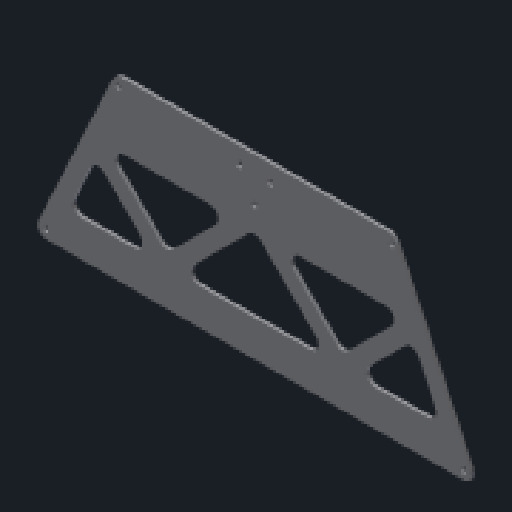
# Autodesk Inventor part: ChestFront
Saved by Autodesk Inventor 2025.2 (Build 292293000, 293)
## iProperties
Created: 2025-02-22
Part Number: ChestFront
Material: Generic
Document SubType Name: Sheet Metal
Designer: valer
Density: 1 g/cm^3
Sheet Metal Rule: Default
Appearance: Default
Author: valer
Autodesk Inventor part; units mm, degrees
ref_plane "YZ Plane" through (0, 0, 0) normal (1, 0, 0) x (0, 1, 0)
ref_plane "XZ Plane" through (0, 0, 0) normal (0, 1, 0) x (-1, 0, 0)
ref_plane "XY Plane" through (0, 0, 0) normal (0, 0, 1) x (1, 0, 0)
sketch "Sketch1" plane through (0, 0, 0) normal (0, 0, 1) x (1, 0, 0)
  line L0 (-64.749, 104.525) -> (-139.8022, 4.926) construction
  line L1 (0, 104.525) -> (-64.749, 104.525) construction
  line L2 (-139.8022, 4.926) -> (-218.9225, -165.525) construction
  line L3 (0, -219.535) -> (0, 158.535) construction
  line L4 (64.749, 104.525) -> (139.8022, 4.926) construction
  line L5 (0, 104.525) -> (64.749, 104.525) construction
  line L6 (139.8022, 4.926) -> (218.9225, -165.525) construction
  line L7 (-218.9225, -165.525) -> (0, -165.525) construction
  line L8 (218.9225, -165.525) -> (0, -165.525) construction
  line L9 (-62.7547, 100.525) -> (-136.3525, 2.8574) construction
  line L10 (-136.3525, 2.8574) -> (-212.6558, -161.525)
  line L11 (-212.6558, -161.525) -> (0, -161.525)
  line L12 (0, -161.525) -> (212.6558, -161.525)
  line L13 (212.6558, -161.525) -> (136.3525, 2.8574)
  line L14 (136.3525, 2.8574) -> (62.7547, 100.525) construction
  line L15 (62.7547, 100.525) -> (0, 100.525) construction
  line L16 (0, 100.525) -> (-62.7547, 100.525) construction
  line L17 (-136.3525, 2.8574) -> (-131.8312, 8.8574)
  line L18 (-131.8312, 8.8574) -> (0, 8.8574)
  line L19 (136.3525, 2.8574) -> (131.8312, 8.8574)
  line L20 (131.8312, 8.8574) -> (0, 8.8574)
  point P0 (0, 0)
  dimension "d0" = 4
  dimension "d34" = 6
  measures "d0" distance between parallel lines of L1 L16
  measures "d34" distance from line of L18 L9.end
extrude "Plate1" add sketch "Sketch1" along normal blind 3.048
fillet "Fillet1" radius 8 6 edges at (-212.6558, -161.525, 1.524) (212.6558, -161.525, 1.524) (-131.8312, 8.8574, 1.524) (-136.3525, 2.8574, 1.524) (131.8312, 8.8574, 1.524) (136.3525, 2.8574, 1.524)
sketch "Sketch3" plane through (0, 0, 3.048) normal (0, 0, 1) x (1, 0, 0)
  arc A0 (200.1225, -161.525) -> (207.3789, -150.1567) centre (200.1225, -153.525) ccw construction
  line L0 (136.7095, 2.0883) -> (207.3789, -150.1567) construction
  line L1 (-207.3789, -150.1567) -> (-136.7095, 2.0883) construction
  arc A1 (-207.3789, -150.1567) -> (-200.1225, -161.525) centre (-200.1225, -153.525) ccw construction
  line L2 (200.1225, -161.525) -> (-200.1225, -161.525) construction
  line L3 (-59.7632, 94.525) -> (59.7632, 94.525) construction
  line L4 (59.7632, 94.525) -> (131.178, -0.2457) construction
  line L5 (131.178, -0.2457) -> (203.2558, -155.525) construction
  line L6 (203.2558, -155.525) -> (-203.2558, -155.525) construction
  line L7 (-203.2558, -155.525) -> (-131.178, -0.2457) construction
  line L8 (-131.178, -0.2457) -> (-59.7632, 94.525) construction
  circle A2 centre (-59.7632, 94.525) radius 3
  circle A3 centre (59.7632, 94.525) radius 3
  circle A4 centre (-131.178, -0.2457) radius 3
  circle A5 centre (131.178, -0.2457) radius 3
  circle A6 centre (-200.1225, -153.525) radius 3
  line L9 (0, -215.7211) -> (0, 149.7327) construction
  circle A7 centre (200.1225, -153.525) radius 3
  arc A8 (136.7095, 2.0883) -> (135.8422, 3.5345) centre (129.4531, -1.28) ccw projected
  line L10 (134.2316, 5.6719) -> (135.8422, 3.5345) projected
  arc A9 (134.2316, 5.6719) -> (127.8425, 8.8574) centre (127.8425, 0.8574) ccw projected
  line L11 (-127.8425, 8.8574) -> (127.8425, 8.8574) projected
  arc A10 (-127.8425, 8.8574) -> (-134.2316, 5.6719) centre (-127.8425, 0.8574) ccw projected
  line L12 (-135.8422, 3.5345) -> (-134.2316, 5.6719) projected
  arc A11 (-135.8422, 3.5345) -> (-136.7095, 2.0883) centre (-129.4531, -1.28) ccw projected
  point P0 (0, 0)
  dimension "d4" = 6
  constraints: 12 end point, 6 centre point, 5 coincident, 4 equal radius, 1 symmetric about line, 3 other
  measures "d4" diameter of A2
extrude "Cut1" cut sketch "Sketch3" against normal blind 3.048
sketch "Sketch5" plane through (0, 0, 3.048) normal (0, 0, 1) x (1, 0, 0)
  circle A0 centre (-131.178, -0.2457) radius 3 construction
  circle A1 centre (131.178, -0.2457) radius 3 construction
  circle A2 centre (-200.1225, -153.525) radius 3 construction
  circle A3 centre (200.1225, -153.525) radius 3 construction
  arc A4 (136.7095, 2.0883) -> (135.8422, 3.5345) centre (129.4531, -1.28) ccw construction
  line L0 (134.2316, 5.6719) -> (135.8422, 3.5345) construction
  arc A5 (134.2316, 5.6719) -> (127.8425, 8.8574) centre (127.8425, 0.8574) ccw construction
  line L1 (-127.8425, 8.8574) -> (127.8425, 8.8574) construction
  arc A6 (-127.8425, 8.8574) -> (-134.2316, 5.6719) centre (-127.8425, 0.8574) ccw construction
  line L2 (-135.8422, 3.5345) -> (-134.2316, 5.6719) construction
  arc A7 (-135.8422, 3.5345) -> (-136.7095, 2.0883) centre (-129.4531, -1.28) ccw construction
  line L3 (-207.3789, -150.1567) -> (-136.7095, 2.0883) construction
  arc A8 (-207.3789, -150.1567) -> (-200.1225, -161.525) centre (-200.1225, -153.525) ccw construction
  line L4 (200.1225, -161.525) -> (-200.1225, -161.525) construction
  arc A9 (200.1225, -161.525) -> (207.3789, -150.1567) centre (200.1225, -153.525) ccw construction
  line L5 (136.7095, 2.0883) -> (207.3789, -150.1567) construction
  line L6 (0, -198.138) -> (0, 44.2342) construction
  line L7 (-100, 8.8574) -> (-100, -161.525) construction
  line L8 (-207.3789, -150.1567) -> (-136.7095, 2.0883) projected
  line L9 (200.1225, -161.525) -> (-200.1225, -161.525) projected
  line L10 (-15, -7.1426) -> (15, -7.1426) construction
  line L11 (15, -7.1426) -> (0, -33.1234) construction
  line L12 (0, -33.1234) -> (-15, -7.1426) construction
  circle A10 centre (-15, -7.1426) radius 3
  circle A11 centre (15, -7.1426) radius 3
  circle A12 centre (0, -33.1234) radius 3
  circle A13 centre (-100, -38.1039) radius 3
  circle A14 centre (-100, -142.6039) radius 3
  circle A15 centre (100, -38.1039) radius 3
  circle A16 centre (100, -142.6039) radius 3
  line L13 (0, -54.1039) -> (-72.5, -126.6039)
  line L14 (-72.5, -126.6039) -> (72.5, -126.6039)
  line L15 (72.5, -126.6039) -> (0, -54.1039)
  line L16 (-84.1532, -115.1039) -> (-23.1532, -54.1039)
  line L17 (-23.1532, -54.1039) -> (-145.1532, -54.1039)
  line L18 (-145.1532, -54.1039) -> (-84.1532, -115.1039)
  line L19 (-152.4933, -69.9169) -> (-95.8064, -126.6039)
  line L20 (-95.8064, -126.6039) -> (-178.8064, -126.6039)
  line L21 (-178.8064, -126.6039) -> (-152.4933, -69.9169)
  line L22 (-145.1532, -54.1039) -> (-152.4933, -69.9169) construction
  line L23 (-23.1532, -54.1039) -> (0, -54.1039) construction
  line L24 (-95.8064, -126.6039) -> (-72.5, -126.6039) construction
  line L25 (-84.1532, -115.1039) -> (-84.1532, -126.6039) construction
  line L26 (84.1532, -115.1039) -> (23.1532, -54.1039)
  line L27 (23.1532, -54.1039) -> (145.1532, -54.1039)
  line L28 (145.1532, -54.1039) -> (84.1532, -115.1039)
  line L29 (152.4933, -69.9169) -> (95.8064, -126.6039)
  line L30 (95.8064, -126.6039) -> (178.8064, -126.6039)
  line L31 (178.8064, -126.6039) -> (152.4933, -69.9169)
  point P0 (0, 0)
  point P1 (0, -7.1426)
  dimension "d38" = 60
  dimension "d39" = 30
  dimension "d40" = 16
  dimension "d41" = 6
  dimension "d54" = 100
  dimension "d57" = 45
  dimension "d58" = 16
  dimension "d59" = 16
  dimension "d60" = 145
  dimension "d61" = 122
  dimension "d62" = 83
  dimension "d63" = 16
  constraints: 46 end point, 8 symmetric about line, 7 centre point, 6 point on line, 5 perpendicular, 4 equal radius, 4 horizontal, 3 coincident, 3 collinear, 3 parallel, 2 midpoint, 1 equal length, 2 other
  measures "d38" angle of L10 L12
  measures "d39" distance of L10.start L10.end
  measures "d40" distance between parallel lines of L1 L10
  measures "d41" diameter of A10
  measures "d54" distance between parallel lines of L6 L7
  measures "d57" angle of L14 L13
  measures "d58" distance from line of L17 A13.centre
  measures "d59" distance from line of L20 A14.centre
  measures "d60" distance of L13.end L14.end
  measures "d61" distance of L16.end L17.end
  measures "d62" distance of L19.end L20.end
  measures "d63" distance between parallel lines of L3 L21
extrude "Cut3" cut sketch "Sketch5" against normal blind 3.048 contours A10 | A11 | A12 | L15 L14 L13 | L18 L17 L16 | L19 L20 L21 | L26 L27 L28 | L31 L30 L29
fillet "Fillet3" radius 8 15 edges at (72.5, -126.6039, 1.524) (0, -54.1039, 1.524) (-72.5, -126.6039, 1.524) (-178.8064, -126.6039, 1.524) (-152.4933, -69.9169, 1.524) (-95.8064, -126.6039, 1.524) (178.8064, -126.6039, 1.524) (95.8064, -126.6039, 1.524) (152.4933, -69.9169, 1.524) (145.1532, -54.1039, 1.524) (84.1532, -115.1039, 1.524) (23.1532, -54.1039, 1.524) (-84.1532, -115.1039, 1.524) (-145.1532, -54.1039, 1.524) (-23.1532, -54.1039, 1.524)
equation "\"d4\" = d3"
equation "\"d5\" = Thickness"
equation "\"d1\" = Thickness"
equation "\"BendRadius\" = Thickness"
equation "\"BendReliefWidth\" = Thickness"
equation "\"BendReliefDepth\" = 0.5 * Thickness"
equation "\"CornerReliefSize\" = 4 * Thickness"
equation "\"MinimumRemnant\" = 2 * Thickness"
equation "\"TransitionRadius\" = BendRadius"
equation "\"JacobiRadiusSize\" = BendRadius"
equation "\"GapSize\" = Thickness"
equation "\"d3\" = 6"
equation "\"Thickness\" = 3.048"
body "Solid1"
